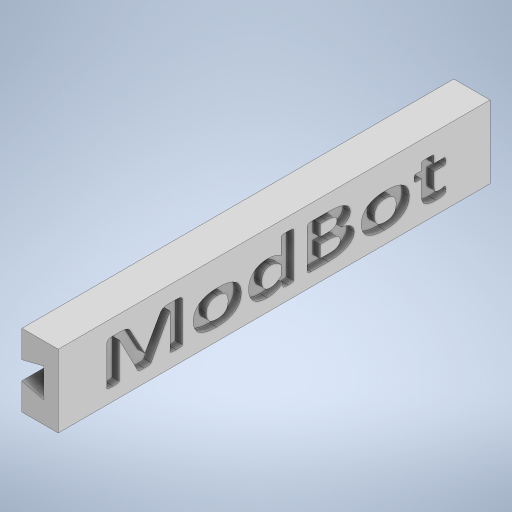
# Autodesk Inventor part: modbot
Saved by Autodesk Inventor 2023 (Build 270158000, 158)
## iProperties
Created: 2024-04-25
Part Number: modbot
Material: Ogólny
Document SubType Name: Modeling
Designer: Kamil
Density: 1 g/cm^3
Appearance: Domyślna
Author: Kamil
Autodesk Inventor part; units mm, degrees
ref_plane "YZ Plane" through (0, 0, 0) normal (1, 0, 0) x (0, 1, 0)
ref_plane "XZ Plane" through (0, 0, 0) normal (0, 1, 0) x (-1, 0, 0)
ref_plane "XY Plane" through (0, 0, 0) normal (0, 0, 1) x (1, 0, 0)
sketch "Szkic1" plane through (0, 0, 0) normal (1, 0, 0) x (0, 1, 0)
  line L0 (6, 56.5) -> (-4, 56.5)
  line L1 (-4, 56.5) -> (-4, -3)
  line L2 (-4, -3) -> (6, -3)
  line L3 (6, -3) -> (6, 56.5)
  point P0 (0, 0)
  dimension "d0" = 10
  dimension "d1" = 59.5
  constraints: 8 end point, 2 parallel, 1 horizontal, 1 perpendicular
  measures "d0" distance of L2.end L1.end
  measures "d1" distance of L1.end L0.end
extrude "Wyciągnięcie proste1" add sketch "Szkic1" against normal blind 5
sketch "Szkic3" plane through (0, -4, -3) normal (0, 0, -1) x (-1, 0, 0)
  line L0 (2, 7) -> (2, 3)
  line L1 (2, 3) -> (5, 3.75)
  line L2 (2, 7) -> (5, 6.25)
  line L3 (5, 6.25) -> (5, 3.75)
  line L4 (5, 10) -> (5, 0) projected
  point P0 (0, 4)
  point P1 (5, 5)
  point P2 (5, 5)
  point P3 (2, 5)
  point P4 (5, 5)
  dimension "d8" = 4
  dimension "d12" = 3
  dimension "d13" = 2.5
  constraints: 10 end point, 4 midpoint, 2 coincident, 1 horizontal alignment, 1 parallel, 1 vertical
  measures "d8" distance of L0.start L0.end
  measures "d12" distance between parallel lines of L3 L0
  measures "d13" distance of L2.end L1.end
extrude "Wyciągnięcie proste3" cut sketch "Szkic3" against normal through all
sketch "Szkic4" plane through (0, 0, 0) normal (1, 0, 0) x (0, 0, -1)
  line L0 (-56.5, -4) -> (3, -4) projected
  line L1 (3, -4) -> (3, 6) projected
  line L2 (3, 6) -> (-56.5, 6) projected
  line L3 (-56.5, 6) -> (-56.5, -4) projected
  line L4 (-51.75, 4.5) -> (-1.75, 4.5) construction
  line L5 (-1.75, 4.5) -> (-1.75, -2.5) construction
  line L6 (-1.75, -2.5) -> (-51.75, -2.5) construction
  line L7 (-51.75, -2.5) -> (-51.75, 4.5) construction
  spline S0 degree 2 poles (-39.381, -1.9831) (-39.381, -2.0338) (-39.4542, -2.107) (-39.657, -2.1521) (-39.9894, -2.1803) (-40.243, -2.1803) knots 0 0 0 1 2 3 4 4 4
  spline S1 degree 2 poles (-40.243, -2.1803) (-40.4908, -2.1803) (-40.8232, -2.1521) (-41.0204, -2.107) (-41.0993, -2.0338) (-41.0993, -1.9831) knots 0 0 0 1 2 3 4 4 4
  line L8 (-41.0993, -1.9831) -> (-41.0993, 2.8732)
  line L9 (-41.0993, 2.8732) -> (-41.1162, 2.8732)
  line L10 (-41.1162, 2.8732) -> (-43.7077, -1.9831)
  spline S2 degree 2 poles (-43.7077, -1.9831) (-43.7359, -2.0394) (-43.8599, -2.1183) (-44.0739, -2.1634) (-44.4063, -2.1803) (-44.643, -2.1803) knots 0 0 0 1 2 3 4 4 4
  spline S3 degree 2 poles (-44.643, -2.1803) (-44.8796, -2.1803) (-45.212, -2.1577) (-45.4261, -2.107) (-45.55, -2.0338) (-45.5669, -1.9831) knots 0 0 0 1 2 3 4 4 4
  line L11 (-45.5669, -1.9831) -> (-48.0739, 2.8732)
  line L12 (-48.0739, 2.8732) -> (-48.0852, 2.8732)
  line L13 (-48.0852, 2.8732) -> (-48.0852, -1.9831)
  spline S4 degree 2 poles (-48.0852, -1.9831) (-48.0852, -2.0338) (-48.1641, -2.107) (-48.3725, -2.1521) (-48.6937, -2.1803) (-48.9528, -2.1803) knots 0 0 0 1 2 3 4 4 4
  spline S5 degree 2 poles (-48.9528, -2.1803) (-49.2007, -2.1803) (-49.5331, -2.1521) (-49.7303, -2.107) (-49.8092, -2.0338) (-49.8092, -1.9831) knots 0 0 0 1 2 3 4 4 4
  line L14 (-49.8092, -1.9831) -> (-49.8092, 3.3352)
  spline S6 degree 2 poles (-49.8092, 3.3352) (-49.8092, 3.5718) (-49.4373, 3.8197) (-49.1218, 3.8197) knots 0 0 0 1 2 2 2
  line L15 (-49.1218, 3.8197) -> (-47.9331, 3.8197)
  spline S7 degree 2 poles (-47.9331, 3.8197) (-47.6176, 3.8197) (-47.1613, 3.7521) (-46.8289, 3.5887) (-46.6092, 3.3296) (-46.5246, 3.1324) knots 0 0 0 1 2 3 4 4 4
  line L16 (-46.5246, 3.1324) -> (-44.5866, -0.4282)
  line L17 (-44.5866, -0.4282) -> (-44.5585, -0.4282)
  line L18 (-44.5585, -0.4282) -> (-42.5528, 3.1268)
  spline S8 degree 2 poles (-42.5528, 3.1268) (-42.4627, 3.3183) (-42.2486, 3.5831) (-41.9669, 3.7521) (-41.5782, 3.8197) (-41.3246, 3.8197) knots 0 0 0 1 2 3 4 4 4
  line L19 (-41.3246, 3.8197) -> (-40.0965, 3.8197)
  spline S9 degree 2 poles (-40.0965, 3.8197) (-39.9106, 3.8197) (-39.6401, 3.7577) (-39.4711, 3.6338) (-39.381, 3.4535) (-39.381, 3.3352) knots 0 0 0 1 2 3 4 4 4
  line L20 (-39.381, 3.3352) -> (-39.381, -1.9831)
  spline S10 degree 2 poles (-31.2908, 0.107) (-31.2908, -0.4225) (-31.7077, -1.2901) (-32.5472, -1.9155) (-33.8204, -2.2592) (-34.6711, -2.2592) knots 0 0 0 1 2 3 4 4 4
  spline S11 degree 2 poles (-34.6711, -2.2592) (-35.4937, -2.2592) (-36.7106, -1.9549) (-37.5162, -1.3746) (-37.9049, -0.5239) (-37.9049, 0.0225) knots 0 0 0 1 2 3 4 4 4
  spline S12 degree 2 poles (-37.9049, 0.0225) (-37.9049, 0.5465) (-37.4824, 1.4197) (-36.6373, 2.0451) (-35.3697, 2.3831) (-34.519, 2.3831) knots 0 0 0 1 2 3 4 4 4
  spline S13 degree 2 poles (-34.519, 2.3831) (-33.6908, 2.3831) (-32.4739, 2.0845) (-31.6796, 1.5042) (-31.2908, 0.6535) (-31.2908, 0.107) knots 0 0 0 1 2 3 4 4 4
  spline S14 degree 2 poles (-33.0824, 0.0563) (-33.0824, 0.3662) (-33.2289, 0.8732) (-33.5725, 1.2563) (-34.1472, 1.4648) (-34.581, 1.4648) knots 0 0 0 1 2 3 4 4 4
  spline S15 degree 2 poles (-34.581, 1.4648) (-34.9697, 1.4648) (-35.55, 1.2789) (-35.9275, 0.9127) (-36.1134, 0.4) (-36.1134, 0.0732) knots 0 0 0 1 2 3 4 4 4
  spline S16 degree 2 poles (-36.1134, 0.0732) (-36.1134, -0.231) (-35.9613, -0.7437) (-35.6232, -1.1211) (-35.0373, -1.3296) (-34.6092, -1.3296) knots 0 0 0 1 2 3 4 4 4
  spline S17 degree 2 poles (-34.6092, -1.3296) (-34.2148, -1.3296) (-33.6345, -1.1437) (-33.2627, -0.7831) (-33.0824, -0.2704) (-33.0824, 0.0563) knots 0 0 0 1 2 3 4 4 4
  spline S18 degree 2 poles (-24.0627, -1.9944) (-24.0627, -2.0451) (-24.1303, -2.1127) (-24.2993, -2.1634) (-24.581, -2.1803) (-24.7894, -2.1803) knots 0 0 0 1 2 3 4 4 4
  spline S19 degree 2 poles (-24.7894, -2.1803) (-25.0092, -2.1803) (-25.2852, -2.1634) (-25.4599, -2.1127) (-25.5331, -2.0451) (-25.5331, -1.9944) knots 0 0 0 1 2 3 4 4 4
  line L21 (-25.5331, -1.9944) -> (-25.5331, -1.538)
  spline S20 degree 2 poles (-25.5331, -1.538) (-26.012, -1.8817) (-27.0542, -2.2592) (-27.6908, -2.2592) knots 0 0 0 1 2 2 2
  spline S21 degree 2 poles (-27.6908, -2.2592) (-28.3951, -2.2592) (-29.3754, -1.893) (-29.9894, -1.2732) (-30.2655, -0.4507) (-30.2655, 0.0056) knots 0 0 0 1 2 3 4 4 4
  spline S22 degree 2 poles (-30.2655, 0.0056) (-30.2655, 0.5577) (-29.9106, 1.4366) (-29.2345, 2.0507) (-28.2261, 2.3831) (-27.5669, 2.3831) knots 0 0 0 1 2 3 4 4 4
  spline S23 degree 2 poles (-27.5669, 2.3831) (-27.0486, 2.3831) (-26.2035, 2.1014) (-25.7923, 1.831) knots 0 0 0 1 2 2 2
  line L22 (-25.7923, 1.831) -> (-25.7923, 4.062)
  spline S24 degree 2 poles (-25.7923, 4.062) (-25.7923, 4.107) (-25.7134, 4.1803) (-25.5162, 4.231) (-25.1838, 4.2592) (-24.9246, 4.2592) knots 0 0 0 1 2 3 4 4 4
  spline S25 degree 2 poles (-24.9246, 4.2592) (-24.6711, 4.2592) (-24.3387, 4.231) (-24.1472, 4.1803) (-24.0627, 4.107) (-24.0627, 4.062) knots 0 0 0 1 2 3 4 4 4
  line L23 (-24.0627, 4.062) -> (-24.0627, -1.9944)
  spline S26 degree 2 poles (-25.7923, 0.7549) (-26.1641, 1.0704) (-26.8514, 1.4028) (-27.2232, 1.4028) knots 0 0 0 1 2 2 2
  spline S27 degree 2 poles (-27.2232, 1.4028) (-27.5613, 1.4028) (-28.0514, 1.1775) (-28.35, 0.8) (-28.4965, 0.3324) (-28.4965, 0.0845) knots 0 0 0 1 2 3 4 4 4
  spline S28 degree 2 poles (-28.4965, 0.0845) (-28.4965, -0.169) (-28.3725, -0.6592) (-28.0852, -1.0423) (-27.6176, -1.2732) (-27.257, -1.2732) knots 0 0 0 1 2 3 4 4 4
  spline S29 degree 2 poles (-27.257, -1.2732) (-27.0768, -1.2732) (-26.7387, -1.2056) (-26.3838, -1.0479) (-26.012, -0.7944) (-25.7923, -0.6085) knots 0 0 0 1 2 3 4 4 4
  line L24 (-25.7923, -0.6085) -> (-25.7923, 0.7549)
  spline S30 degree 2 poles (-15.7303, -0.3606) (-15.7303, -0.6817) (-15.9894, -1.1944) (-16.457, -1.5944) (-17.0993, -1.8817) (-17.8711, -2.062) (-18.75, -2.1521) (-19.2908, -2.1521) knots 0 0 0 1 2 3 4 5 6 6 6
  line L25 (-19.2908, -2.1521) -> (-21.6683, -2.1521)
  spline S31 degree 2 poles (-21.6683, -2.1521) (-21.8993, -2.1521) (-22.2092, -1.9718) (-22.2092, -1.769) knots 0 0 0 1 2 2 2
  line L26 (-22.2092, -1.769) -> (-22.2092, 3.4366)
  spline S32 degree 2 poles (-22.2092, 3.4366) (-22.2092, 3.6394) (-21.8993, 3.8197) (-21.6683, 3.8197) knots 0 0 0 1 2 2 2
  line L27 (-21.6683, 3.8197) -> (-19.4204, 3.8197)
  spline S33 degree 2 poles (-19.4204, 3.8197) (-18.5979, 3.8197) (-17.4599, 3.6338) (-16.6768, 3.262) (-16.2599, 2.6873) (-16.2599, 2.3042) knots 0 0 0 1 2 3 4 4 4
  spline S34 degree 2 poles (-16.2599, 2.3042) (-16.2599, 2.0845) (-16.4289, 1.7014) (-16.7444, 1.3859) (-17.2063, 1.1493) (-17.5049, 1.0761) knots 0 0 0 1 2 3 4 4 4
  spline S35 degree 2 poles (-17.5049, 1.0761) (-17.1275, 1.031) (-16.4852, 0.8) (-16.0063, 0.4338) (-15.7303, -0.0563) (-15.7303, -0.3606) knots 0 0 0 1 2 3 4 4 4
  spline S36 degree 2 poles (-17.6176, -0.4) (-17.6176, -0.1972) (-17.8261, 0.1352) (-18.2261, 0.3549) (-18.8458, 0.4732) (-19.3472, 0.4732) knots 0 0 0 1 2 3 4 4 4
  line L28 (-19.3472, 0.4732) -> (-20.4232, 0.4732)
  line L29 (-20.4232, 0.4732) -> (-20.4232, -1.2225)
  line L30 (-20.4232, -1.2225) -> (-19.1106, -1.2225)
  spline S37 degree 2 poles (-19.1106, -1.2225) (-18.7275, -1.2225) (-18.2092, -1.1155) (-17.8317, -0.9127) (-17.6176, -0.6028) (-17.6176, -0.4) knots 0 0 0 1 2 3 4 4 4
  spline S38 degree 2 poles (-18.0796, 2.1521) (-18.0796, 2.3324) (-18.2486, 2.6197) (-18.5754, 2.8113) (-19.0824, 2.9127) (-19.5049, 2.9127) knots 0 0 0 1 2 3 4 4 4
  line L31 (-19.5049, 2.9127) -> (-20.4232, 2.9127)
  line L32 (-20.4232, 2.9127) -> (-20.4232, 1.3634)
  line L33 (-20.4232, 1.3634) -> (-19.4092, 1.3634)
  spline S39 degree 2 poles (-19.4092, 1.3634) (-19.0148, 1.3634) (-18.5415, 1.4873) (-18.2317, 1.7014) (-18.0796, 1.9944) (-18.0796, 2.1521) knots 0 0 0 1 2 3 4 4 4
  spline S40 degree 2 poles (-8.1359, 0.107) (-8.1359, -0.4225) (-8.5528, -1.2901) (-9.3923, -1.9155) (-10.6655, -2.2592) (-11.5162, -2.2592) knots 0 0 0 1 2 3 4 4 4
  spline S41 degree 2 poles (-11.5162, -2.2592) (-12.3387, -2.2592) (-13.5556, -1.9549) (-14.3613, -1.3746) (-14.75, -0.5239) (-14.75, 0.0225) knots 0 0 0 1 2 3 4 4 4
  spline S42 degree 2 poles (-14.75, 0.0225) (-14.75, 0.5465) (-14.3275, 1.4197) (-13.4824, 2.0451) (-12.2148, 2.3831) (-11.3641, 2.3831) knots 0 0 0 1 2 3 4 4 4
  spline S43 degree 2 poles (-11.3641, 2.3831) (-10.5359, 2.3831) (-9.319, 2.0845) (-8.5246, 1.5042) (-8.1359, 0.6535) (-8.1359, 0.107) knots 0 0 0 1 2 3 4 4 4
  spline S44 degree 2 poles (-9.9275, 0.0563) (-9.9275, 0.3662) (-10.0739, 0.8732) (-10.4176, 1.2563) (-10.9923, 1.4648) (-11.4261, 1.4648) knots 0 0 0 1 2 3 4 4 4
  spline S45 degree 2 poles (-11.4261, 1.4648) (-11.8148, 1.4648) (-12.3951, 1.2789) (-12.7725, 0.9127) (-12.9585, 0.4) (-12.9585, 0.0732) knots 0 0 0 1 2 3 4 4 4
  spline S46 degree 2 poles (-12.9585, 0.0732) (-12.9585, -0.231) (-12.8063, -0.7437) (-12.4683, -1.1211) (-11.8824, -1.3296) (-11.4542, -1.3296) knots 0 0 0 1 2 3 4 4 4
  spline S47 degree 2 poles (-11.4542, -1.3296) (-11.0599, -1.3296) (-10.4796, -1.1437) (-10.1077, -0.7831) (-9.9275, -0.2704) (-9.9275, 0.0563) knots 0 0 0 1 2 3 4 4 4
  spline S48 degree 2 poles (-3.1049, -1.5887) (-3.1049, -1.7915) (-3.1838, -2.0113) (-3.3077, -2.0958) (-3.55, -2.1634) (-3.8711, -2.2141) (-4.2542, -2.2423) (-4.4458, -2.2423) knots 0 0 0 1 2 3 4 5 6 6 6
  spline S49 degree 2 poles (-4.4458, -2.2423) (-4.9641, -2.2423) (-5.7246, -2.0676) (-6.2261, -1.707) (-6.4627, -1.1493) (-6.4627, -0.7718) knots 0 0 0 1 2 3 4 4 4
  line L34 (-6.4627, -0.7718) -> (-6.4627, 1.3352)
  line L35 (-6.4627, 1.3352) -> (-7.2007, 1.3352)
  spline S50 degree 2 poles (-7.2007, 1.3352) (-7.3303, 1.3352) (-7.4711, 1.5549) (-7.4711, 1.8085) knots 0 0 0 1 2 2 2
  spline S51 degree 2 poles (-7.4711, 1.8085) (-7.4711, 1.9437) (-7.4373, 2.1296) (-7.3641, 2.231) (-7.2627, 2.2817) (-7.1951, 2.2817) knots 0 0 0 1 2 3 4 4 4
  line L36 (-7.1951, 2.2817) -> (-6.4627, 2.2817)
  line L37 (-6.4627, 2.2817) -> (-6.4627, 3.2)
  spline S52 degree 2 poles (-6.4627, 3.2) (-6.4627, 3.2451) (-6.3838, 3.3183) (-6.181, 3.369) (-5.843, 3.3915) (-5.5951, 3.3915) knots 0 0 0 1 2 3 4 4 4
  spline S53 degree 2 poles (-5.5951, 3.3915) (-5.3415, 3.3915) (-5.0035, 3.369) (-4.8063, 3.3183) (-4.7218, 3.2451) (-4.7218, 3.2) knots 0 0 0 1 2 3 4 4 4
  line L38 (-4.7218, 3.2) -> (-4.7218, 2.2817)
  line L39 (-4.7218, 2.2817) -> (-3.381, 2.2817)
  spline S54 degree 2 poles (-3.381, 2.2817) (-3.3134, 2.2817) (-3.212, 2.231) (-3.1387, 2.1296) (-3.1049, 1.9437) (-3.1049, 1.8085) knots 0 0 0 1 2 3 4 4 4
  spline S55 degree 2 poles (-3.1049, 1.8085) (-3.1049, 1.5549) (-3.2458, 1.3352) (-3.3754, 1.3352) knots 0 0 0 1 2 2 2
  line L40 (-3.3754, 1.3352) -> (-4.7218, 1.3352)
  line L41 (-4.7218, 1.3352) -> (-4.7218, -0.5972)
  spline S56 degree 2 poles (-4.7218, -0.5972) (-4.7218, -0.9352) (-4.4063, -1.2676) (-4.0007, -1.2676) knots 0 0 0 1 2 2 2
  spline S57 degree 2 poles (-4.0007, -1.2676) (-3.8599, -1.2676) (-3.6401, -1.2394) (-3.4655, -1.1944) (-3.3472, -1.1662) (-3.3021, -1.1662) knots 0 0 0 1 2 3 4 4 4
  spline S58 degree 2 poles (-3.3021, -1.1662) (-3.257, -1.1662) (-3.1838, -1.1944) (-3.1387, -1.2958) (-3.1049, -1.4592) (-3.1049, -1.5887) knots 0 0 0 1 2 3 4 4 4
  point P0 (0, 0)
  point P1 (-51.75, 1)
  point P2 (-56.5, 1)
  point P3 (-26.75, 4.5)
  point P4 (-26.75, 6)
  dimension "d18" = 50
  dimension "d19" = 7
  constraints: 4 midpoint, 1 horizontal alignment, 1 vertical alignment, 2 other
  measures "d18" distance of L5.end L6.end
  measures "d19" distance between parallel lines of L6 L4
extrude "Wyciągnięcie proste4" cut sketch "Szkic4" against normal blind 1 contours S0 S1 L8 L9 L10 S2 S3 L11 L12 L13 S4 S5 L14 S6 L15 S7 L16 L17 L18 S8 L19 S9 L20 | S10 S11 S12 S13 | S18 S19 L21 S20 S21 S22 S23 L22 S24 S25 L23 | S30 L25 S31 L26 S32 L27 S33 S34 S35 | S40 S41 S42 S43 | S48 S49 L34 L35 S50 S51 L36 L37 S52 S53 L38 L39 S54 S55 L40 L41 S56 S57 S58
